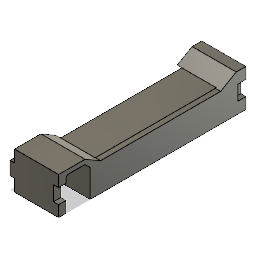
Key v13 (Autodesk Fusion 360 design; units mm, degrees)
Autodesk Fusion 360 part; units mm, degrees
sketch "Sketch1" plane through (0, 0, 0) normal (0, 1, 0) x (1, 0, 0)
  line L0 (14.75, 62.5) -> (-14.75, 62.5)
  line L1 (-14.75, 62.5) -> (-14.75, -62.5)
  line L2 (-14.75, -62.5) -> (14.75, -62.5)
  line L3 (14.75, -62.5) -> (14.75, 62.5)
  line L4 (14.75, 62.5) -> (-14.75, -62.5) construction
  line L5 (-14.75, 62.5) -> (14.75, -62.5) construction
  dimension "d1" = 29.5
  dimension "d4" = 125
  constraint perpendicular L0 L1
  constraint parallel L0 L2
  constraint parallel L1 L3
  constraint horizontal L0
  constraint coincident L4 origin
  constraint coincident L5 origin
  measures "d1" distance of L1.end L2.end
  measures "d4" distance of L0.end L1.end
extrude "Extrude1" add sketch "Sketch1" along normal blind 25
sketch "Sketch2" plane through (14.75, 0, 0) normal (1, 0, 0) x (0, 0, -1)
  line L0 (-62.5, 0) -> (62.5, 0)
  line L1 (62.5, 25) -> (-62.5, 25)
  line L2 (-62.5, 25) -> (-62.5, 0)
  line L3 (-57.5, 0) -> (-41.5, 0)
  line L4 (-41.5, 0) -> (-41.5, 22)
  line L5 (-41.5, 22) -> (-57.5, 22)
  line L6 (-57.5, 22) -> (-57.5, 0)
  dimension "d5" = 16
  dimension "d6" = 5
  dimension "d70" = 3
  constraint horizontal L3
  constraint vertical L4
  constraint horizontal L5
  constraint vertical L6
  constraint coincident L0 L3.start
  measures "d5" distance of L4.end L5.end
  measures "d6" distance of L2 L6
  measures "d70" distance of L1 L5
extrude "Extrude2" cut sketch "Sketch2" against normal through all
sketch "Sketch3" plane through (-14.75, 0, 0) normal (-1, 0, 0) x (0, 0, 1)
  line L0 (57.5, 22) -> (57.5, 0)
  line L1 (57.5, 0) -> (62.5, 0)
  line L2 (62.5, 0) -> (62.5, 25)
  line L3 (62.5, 25) -> (-62.5, 25)
  line L4 (-62.5, 25) -> (-62.5, 0)
  line L5 (-62.5, 0) -> (41.5, 0)
  line L6 (41.5, 0) -> (41.5, 22)
  line L7 (41.5, 22) -> (57.5, 22)
  line L8 (-57.5, 0) -> (37.5, 0)
  line L9 (37.5, 0) -> (37.5, 14.5)
  line L10 (37.5, 14.5) -> (-57.5, 14.5)
  line L11 (-57.5, 14.5) -> (-57.5, 0)
  dimension "d12" = 4
  dimension "d51" = 5
  dimension "d69" = 10.5
  constraint horizontal L8
  constraint vertical L9
  constraint horizontal L10
  constraint vertical L11
  constraint collinear L5 L8
  measures "d12" distance of L6 L9
  measures "d51" distance of L4 L11
  measures "d69" distance of L3 L10
extrude "Extrude3" cut sketch "Sketch3" against normal blind 26 contours L5 L8 L9 L10 L11
sketch "Sketch4" plane through (-14.75, 0, 0) normal (-1, 0, 0) x (0, 0, 1)
  line L0 (37.5, 14.5) -> (37.5, 0)
  line L1 (37.5, 0) -> (41.5, 0)
  line L2 (41.5, 0) -> (41.5, 22)
  line L3 (41.5, 22) -> (57.5, 22)
  line L4 (57.5, 22) -> (57.5, 0)
  line L5 (57.5, 0) -> (62.5, 0)
  line L6 (62.5, 0) -> (62.5, 25)
  line L7 (62.5, 25) -> (-62.5, 25)
  line L8 (-62.5, 25) -> (-62.5, 0)
  line L9 (-62.5, 0) -> (-57.5, 0)
  line L10 (-57.5, 14.5) -> (37.5, 14.5)
  line L11 (-55.8923, 25) -> (-45.5, 19)
  line L12 (-45.5, 19) -> (34.5, 19)
  line L13 (34.5, 19) -> (44.8923, 25)
  line L14 (-57.5, 0) -> (-57.5, 14.5)
  dimension "d16" = 6
  dimension "d44" = 150
  dimension "d45" = 150
  dimension "d46" = 80
  dimension "d49" = 28
  constraint coincident L7 L11.start
  constraint parallel L7 L12
  constraint coincident L7 L13.end
  measures "d16" vertical distance of L11.start L11.end
  measures "d44" angle of L11 L12
  measures "d45" angle of L12 L13
  measures "d46" distance of L11.end L12.end
  measures "d49" distance of L6 L12.end
extrude "Extrude4" cut sketch "Sketch4" against normal through all contours L7 L11 L12 L13
sketch "Sketch5" plane through (-14.75, 0, 0) normal (-1, 0, 0) x (0, 0, 1)
  line L0 (44.8923, 25) -> (34.5, 19)
  line L1 (34.5, 19) -> (-45.5, 19)
  line L2 (-45.5, 19) -> (-55.8923, 25)
  line L3 (-62.5, 25) -> (-62.5, 0)
  line L4 (-62.5, 0) -> (-57.5, 0)
  line L5 (-57.5, 14.5) -> (37.5, 14.5)
  line L6 (37.5, 14.5) -> (37.5, 0)
  line L7 (37.5, 0) -> (41.5, 0)
  line L8 (41.5, 0) -> (41.5, 22)
  line L9 (-50.5, 19) -> (39.5, 19)
  line L10 (39.5, 19) -> (39.5, 16.05)
  line L11 (39.5, 16.05) -> (-50.5, 16.05)
  line L12 (-50.5, 16.05) -> (-50.5, 19)
  line L13 (-57.5, 0) -> (-57.5, 14.5)
  line L14 (41.5, 22) -> (57.5, 22)
  line L15 (57.5, 22) -> (57.5, 0)
  line L16 (57.5, 0) -> (62.5, 0)
  line L17 (62.5, 0) -> (62.5, 25)
  line L18 (-55.8923, 25) -> (-62.5, 25)
  line L19 (62.5, 25) -> (44.8923, 25)
  dimension "d21" = 5
  dimension "d22" = 2.95
  dimension "d48" = 5
  constraint horizontal L9
  constraint vertical L10
  constraint horizontal L11
  constraint vertical L12
  constraint collinear L1 L9
  measures "d21" distance of L1.end L12
  measures "d22" distance of L9.start L11.end
  measures "d48" distance of L0.end L9.end
extrude "Extrude5" cut sketch "Sketch5" against normal blind 26 contours L1 L9 L10 L11 L12
sketch "Sketch14" plane through (-14.75, 0, 0) normal (-1, 0, 0) x (0, 0, 1)
  line L0 (34.5, 19) -> (39.5, 19)
  line L1 (39.5, 19) -> (39.5, 16.05)
  line L2 (39.5, 16.05) -> (-50.5, 16.05)
  line L3 (-50.5, 16.05) -> (-50.5, 19)
  line L4 (-50.5, 19) -> (-45.5, 19)
  line L5 (-45.5, 19) -> (-55.8923, 25)
  line L6 (-55.8923, 25) -> (-62.5, 25)
  line L7 (-62.5, 25) -> (-62.5, 0)
  line L8 (-62.5, 0) -> (-57.5, 0)
  line L9 (-57.5, 0) -> (-57.5, 14.5)
  line L10 (-57.5, 14.5) -> (37.5, 14.5)
  line L11 (37.5, 14.5) -> (37.5, 0)
  line L12 (37.5, 0) -> (41.5, 0)
  line L13 (41.5, 0) -> (41.5, 22)
  line L14 (41.5, 22) -> (57.5, 22)
  line L15 (57.5, 22) -> (57.5, 0)
  line L16 (57.5, 0) -> (62.5, 0)
  line L17 (62.5, 0) -> (62.5, 25)
  line L18 (62.5, 25) -> (44.8923, 25)
  line L19 (44.8923, 25) -> (34.5, 19)
  line L20 (-50.5, 19) -> (39.5, 19)
  line L21 (39.5, 19) -> (39.5, 19.25)
  line L22 (39.5, 19.25) -> (-50.5, 19.25)
  line L23 (-50.5, 19.25) -> (-50.5, 19)
  dimension "d90" = 0.25
  constraint horizontal L20
  constraint vertical L21
  constraint horizontal L22
  constraint vertical L23
  constraint coincident L3.end L4.start
  constraint collinear L1 L21
  measures "d90" distance of L20 L22
extrude "Extrude14" cut sketch "Sketch14" against normal up to surface (26 mm away) contours L0 L19 L20 L21 L22 | L4 L5 L20 L22 L23
ref_plane "WorkPlane1" through (0, 12.5, 0) normal (0, 0, -1) x (-1, 0, 0)
sketch "Sketch6" plane through (0, 0, -62.5) normal (0, 0, -1) x (-1, 0, 0)
  line L0 (-14.75, 0) -> (14.75, 0)
  line L1 (14.75, 0) -> (14.75, 25)
  line L2 (-14.75, 25) -> (-14.75, 0)
  line L3 (14.75, 25) -> (-14.75, 25)
  line L4 (14.75, 17) -> (14.75, 8)
  line L5 (14.75, 8) -> (17.75, 8)
  line L6 (17.75, 8) -> (17.75, 17)
  line L7 (17.75, 17) -> (14.75, 17)
  line L8 (17.75, 12.5) -> (14.75, 12.5) construction
  dimension "d52" = 8
  dimension "d53" = 8
  dimension "d54" = 3
  constraint coincident L1 L4.start
  constraint coincident L1 L4.end
  constraint perpendicular L3 L4
  constraint parallel L1 L6
  constraint midpoint L6 L8.start
  constraint midpoint L4 L8.end
  constraint horizontal L8
  constraint horizontal L7
  measures "d52" distance of L0 L4.end
  measures "d53" distance of L3 L4.start
  measures "d54" distance of L4 L6
sketch "Sketch7" plane through (0, 0, -62.5) normal (0, 0, -1) x (-1, 0, 0)
  line L0 (14.75, 0) -> (-14.75, 0)
  line L1 (-14.75, 0) -> (-14.75, 25)
  line L2 (-14.75, 17) -> (-14.75, 8)
  line L3 (-14.75, 8) -> (-11.75, 8)
  line L4 (-14.75, 17) -> (-11.75, 17)
  line L5 (-11.75, 17) -> (-11.75, 8)
  line L6 (-11.75, 12.5) -> (-14.75, 12.5) construction
  dimension "d56" = 8
  dimension "d57" = 8
  dimension "d58" = 3
  constraint coincident L1 L2.start
  constraint coincident L1 L2.end
  constraint midpoint L5 L6.start
  constraint midpoint L2 L6.end
  constraint horizontal L6
  constraint horizontal L4
  measures "d56" distance of L0.end L2.end
  measures "d57" distance of L1.end L2.start
  measures "d58" distance of L2 L5
extrude "Extrude6" add sketch "Sketch6" against normal blind 5 contours L1 L4 L5 L6 L7
extrude "Extrude7" cut sketch "Sketch7" against normal blind 5.5
mirror "Mirror1" about plane through (0, 12.5, 0) normal (0, 0, -1) of "Extrude6", "Extrude7"
sketch "Sketch9" plane through (0, 0, 41.5) normal (0, 0, 1) x (1, 0, 0)
  line L0 (-14.75, 22) -> (-14.75, 0)
  line L1 (-14.75, 0) -> (14.75, 0)
  line L2 (14.75, 0) -> (14.75, 22)
  line L3 (1.25, 20.05) -> (-4.75, 20.05)
  line L4 (-4.75, 20.05) -> (-4.75, 14.05)
  line L5 (-4.75, 14.05) -> (1.25, 14.05)
  line L6 (1.25, 14.05) -> (1.25, 20.05)
  line L7 (1.25, 20.05) -> (-4.75, 14.05) construction
  line L8 (-4.75, 20.05) -> (1.25, 14.05) construction
  line L9 (-14.75, 16.05) -> (11.25, 16.05) construction
  line L10 (-1.75, 16.05) -> (-1.75, 17.05) construction
  line L11 (14.75, 22) -> (-14.75, 22)
  point P0 (-1.75, 17.05)
  dimension "d39" = 6
  dimension "d67" = 4
  constraint perpendicular L3 L4
  constraint parallel L3 L5
  constraint parallel L4 L6
  constraint horizontal L3
  constraint coincident L7 P0
  constraint coincident L8 P0
  constraint midpoint L9 L10.start
  constraint coincident P0 L10.end
  constraint vertical L10
  constraint equal L3 L6
  measures "d39" distance of L3.start L3.end
  measures "d67" distance of L3 L9
extrude "Extrude9" cut sketch "Sketch9" against normal blind 2 contours L3 L4 L5 L6
sketch "Sketch10" plane through (0, 0, -62.5) normal (0, 0, -1) x (-1, 0, 0)
  line L0 (-11.75, 8) -> (-14.75, 8)
  line L1 (-14.75, 8) -> (-14.75, 0)
  line L2 (-14.75, 0) -> (14.75, 0)
  line L3 (14.75, 0) -> (14.75, 8)
  line L4 (14.75, 8) -> (17.75, 8)
  line L5 (17.75, 8) -> (17.75, 17)
  line L6 (17.75, 17) -> (14.75, 17)
  line L7 (14.75, 17) -> (14.75, 25)
  line L8 (14.75, 25) -> (-14.75, 25)
  line L9 (-14.75, 25) -> (-14.75, 17)
  line L10 (-14.75, 17) -> (-11.75, 17)
  line L11 (-11.75, 17) -> (-11.75, 8)
  circle A0 centre (1.75, 8) radius 2
  line L12 (14.75, 14.5) -> (-11.25, 14.5)
  line L13 (1.75, 8) -> (1.75, 14.5) construction
  dimension "d60" = 4
  dimension "d61" = 8
  constraint coincident A0.centre L13.start
  constraint midpoint L12 L13.end
  constraint perpendicular L12 L13
  measures "d60" diameter of A0
  measures "d61" distance of L2 A0.centre
extrude "Extrude10" cut sketch "Sketch10" against normal blind 5 contours A0
fillet "Fillet3" radius 1.5 2 edges at (0, 22, 41.5) (0, 22, 57.5)
sketch "Sketch11" plane through (0, 0, 41.5) normal (0, 0, 1) x (1, 0, 0)
  line L0 (14.75, 20.5) -> (-14.75, 20.5)
  line L1 (-14.75, 20.5) -> (-14.75, 0)
  line L2 (-14.75, 0) -> (14.75, 0)
  line L3 (14.75, 0) -> (14.75, 20.5)
  line L4 (-4.75, 20.05) -> (1.25, 20.05)
  line L5 (1.25, 20.05) -> (1.25, 14.05)
  line L6 (1.25, 14.05) -> (-4.75, 14.05)
  line L7 (-4.75, 14.05) -> (-4.75, 20.05)
  line L8 (-6.95, 18.55) -> (-4.75, 18.55)
  line L9 (-4.75, 18.55) -> (-4.75, 15.55)
  line L10 (-4.75, 15.55) -> (-6.95, 15.55)
  line L11 (-6.95, 15.55) -> (-6.95, 18.55)
  line L12 (3.45, 18.55) -> (1.25, 18.55)
  line L13 (1.25, 18.55) -> (1.25, 15.55)
  line L14 (1.25, 15.55) -> (3.45, 15.55)
  line L15 (3.45, 15.55) -> (3.45, 18.55)
  line L16 (-1.75, 20.05) -> (-1.75, 14.05) construction
  line L17 (-1.75, 17.05) -> (-6.95, 17.05) construction
  dimension "d75" = 2.2
  dimension "d76" = 3
  constraint horizontal L8
  constraint vertical L9
  constraint horizontal L10
  constraint vertical L11
  constraint coincident L7 L9.end
  constraint horizontal L12
  constraint vertical L13
  constraint horizontal L14
  constraint vertical L15
  constraint coincident L5 L13.end
  constraint collinear L10 L14
  constraint collinear L8 L12
  constraint midpoint L4 L16.start
  constraint midpoint L6 L16.end
  constraint midpoint L16 L17.start
  constraint midpoint L11 L17.end
  constraint horizontal L17
  constraint equal L10 L14
  measures "d75" distance of L8.start L8.end
  measures "d76" distance of L8.start L10.end
extrude "Extrude11" cut sketch "Sketch11" against normal up to surface (2 mm away) contours L4 L5 L6 L7 L9 L13 | L7 L8 L9 L10 L11 | L5 L12 L13 L14 L15
fillet "Fillet4" radius 0.5 4 edges at (3.45, 18.55, 40.5) (3.45, 15.55, 40.5) (-6.95, 18.55, 40.5) (-6.95, 15.55, 40.5)
sketch "Sketch12" plane through (14.75, 0, 0) normal (1, 0, 0) x (0, 0, -1)
  line L0 (-62.5, 17) -> (-57.5, 17)
  line L1 (-57.5, 17) -> (-57.5, 20.5)
  arc A0 (-56, 22) -> (-57.5, 20.5) centre (-56, 20.5) ccw
  line L2 (-56, 22) -> (-43, 22)
  arc A1 (-41.5, 20.5) -> (-43, 22) centre (-43, 20.5) ccw
  line L3 (-41.5, 20.5) -> (-41.5, 0)
  line L4 (-41.5, 0) -> (62.5, 0)
  line L5 (62.5, 0) -> (62.5, 8)
  line L6 (62.5, 8) -> (57, 8)
  line L7 (57, 8) -> (57, 17)
  line L8 (57, 17) -> (62.5, 17)
  line L9 (62.5, 17) -> (62.5, 25)
  line L10 (62.5, 25) -> (55.8923, 25)
  line L11 (55.8923, 25) -> (45.5, 19)
  line L12 (45.5, 19) -> (-34.5, 19)
  line L13 (-34.5, 19) -> (-44.8923, 25)
  line L14 (-44.8923, 25) -> (-62.5, 25)
  line L15 (-62.5, 25) -> (-62.5, 17)
  line L16 (-41.5, 18.5) -> (-45, 22)
  dimension "d79" = 3.5
  dimension "d80" = 3.5
  constraint coincident L3 L16.start
  constraint coincident L2 L16.end
  measures "d79" distance of L2 L16.start
  measures "d80" distance of L3 L16.end
extrude "Extrude12" add sketch "Sketch12" against normal blind 4 contours L2 A1 L3 L16
sketch "Sketch13" plane through (0, 0, 62.5) normal (0, 0, 1) x (1, 0, 0)
  line L0 (14.75, 8) -> (11.75, 8)
  line L1 (11.75, 8) -> (11.75, 17)
  line L2 (11.75, 17) -> (14.75, 17)
  line L3 (14.75, 17) -> (14.75, 25)
  line L4 (14.75, 25) -> (-14.75, 25)
  line L5 (-14.75, 25) -> (-14.75, 17)
  line L6 (-14.75, 17) -> (-17.75, 17)
  line L7 (-17.75, 17) -> (-17.75, 8)
  line L8 (-17.75, 8) -> (-14.75, 8)
  line L9 (-14.75, 8) -> (-14.75, 0)
  line L10 (-14.75, 0) -> (14.75, 0)
  line L11 (14.75, 0) -> (14.75, 8)
  line L12 (14.75, 17.4) -> (11.35, 17.4)
  line L13 (11.35, 17.4) -> (11.35, 7.6)
  line L14 (11.35, 7.6) -> (14.75, 7.6)
  dimension "d83" = 0.4
  dimension "d84" = 0.4
  dimension "d85" = 0.4
  constraint coincident L3 L12.start
  constraint parallel L1 L13
  constraint coincident L11 L14.end
  constraint parallel L0 L14
  constraint parallel L2 L12
  measures "d83" distance of L2 L12
  measures "d84" distance of L0 L14
  measures "d85" distance of L1 L13
extrude "Extrude13" cut sketch "Sketch13" against normal blind 5.5 contours L0 L1 L2 L3 L11 L12 L13 L14
mirror "Mirror2" about plane through (0, 0, 0) normal (0, 0, 1) of "Extrude13"
